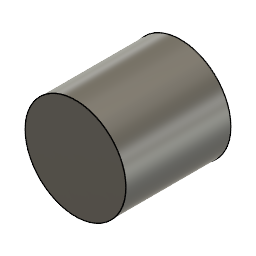
replay (Autodesk Fusion 360 design; units mm, degrees)
Autodesk Fusion 360 part; units mm, degrees
ref_plane "工作平面1" through (0, 0, -19) normal (0, 0, 1) x (1, 0, 0)
sketch "草图1" plane through (0, 0, -19) normal (0, 0, 1) x (1, 0, 0)
  circle A0 centre (18, 10) radius 12
extrude "拉伸1" add sketch "草图1" along normal blind 25
